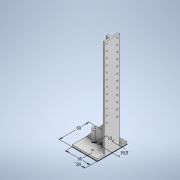
# Autodesk Inventor part: camera arm
Saved by Autodesk Inventor 2021 (Build 250183000, 183)
## iProperties
Created: 2022-11-09
Part Number: camera arm
Material: Generic
Document SubType Name: Modeling
Designer: marti
Density: 1 g/cm^3
Appearance: Default
Author: marti
Autodesk Inventor part; units mm, degrees
ref_plane "YZ Plane" through (0, 0, 0) normal (1, 0, 0) x (0, 1, 0)
ref_plane "XZ Plane" through (0, 0, 0) normal (0, 1, 0) x (-1, 0, 0)
ref_plane "XY Plane" through (0, 0, 0) normal (0, 0, 1) x (1, 0, 0)
sketch "Sketch1" plane through (0, 0, 0) normal (0, 1, 0) x (-1, 0, 0)
  line L0 (-15, -19.5) -> (-15, 0) construction
  line L1 (-15, 0) -> (-15, 19.5) construction
  line L2 (15, -30) -> (-35, -30)
  line L3 (-35, -30) -> (-35, 30)
  line L4 (-35, 30) -> (15, 30)
  line L5 (15, 30) -> (15, -30)
  circle A0 centre (0, 0) radius 5
  point P0 (15, 0)
  dimension "d0" = 15
  dimension "d1" = 19.5
  dimension "d2" = 60
  dimension "d3" = 50
  dimension "d4" = 20
  dimension "d22" = 10
  constraints: 12 end point, 3 equal length, 2 coincident, 2 horizontal alignment, 1 centre point, 1 collinear, 1 horizontal, 1 midpoint, 1 perpendicular, 1 vertical
  measures "d0" horizontal distance of L0.start point (0, 0)
  measures "d1" vertical distance of point (0, 0) L0.start
  measures "d2" distance of L4.end L2.start
  measures "d3" distance of L3.end L4.end
  measures "d4" distance from line of L1.end L3
  measures "d22" diameter of A0
extrude "Extrusion1" add sketch "Sketch1" along normal blind 4 contours L2 L3 L4 L5 | A0
sketch "Sketch2" plane through (0, 0, 0) normal (0, 0, 1) x (1, 0, 0)
  line L0 (35, 4) -> (-15, 4) projected
  line L1 (35, 4) -> (35, 200)
  line L2 (35, 200) -> (25, 200)
  line L3 (25, 200) -> (25, 49)
  line L4 (25, 49) -> (-15, 4)
  line L5 (32, 200) -> (32, 4)
  line L6 (-15, 0) -> (35, 0) projected
  point P0 (0, 0)
  dimension "d14" = 10
  dimension "d15" = 3
  dimension "d16" = 45
  dimension "d17" = 200
  constraints: 10 end point, 3 perpendicular, 2 point on line, 1 vertical
  measures "d14" distance between parallel lines of L3 L1
  measures "d15" distance between parallel lines of L1 L5
  measures "d16" distance from line of L0 L3.end
  measures "d17" distance from line of L6 L5.start
extrude "Extrusion2" add sketch "Sketch2" along normal mid plane 4 contours L0 L4 L3 L2 L5
extrude "breedte arm" add sketch "Sketch2" along normal mid plane 30 contours L0 L5 L2 L1
extrude "Extrusion4" add sketch "Sketch1" along normal blind 25 contours A0
hole "Hole2" at (0, 0, 0) at (15, 0, -19.5) at (15, 0, 19.5) direction (0, 1, 0) diameter 3.4 end through all clearance for "Hex Head Cap Screw ISO 24017" size "M3" standard "ISO"
sketch "Sketch3" plane through (35, 0, 30) normal (1, 0, 0) x (0, 0, -1)
  line L0 (15, 200) -> (45, 200) projected
  line L1 (19.5, 195) -> (15, 195) construction
  line L2 (15, 200) -> (15, 4) construction
  line L3 (40.5, 195) -> (45, 195) construction
  line L4 (45, 4) -> (45, 200) construction
  point P0 (30, 0)
  point P1 (42.75, 195)
  point P2 (19.5, 182.5)
  point P3 (40.5, 182.5)
  point P4 (19.5, 170)
  point P5 (40.5, 170)
  point P6 (19.5, 157.5)
  point P7 (40.5, 157.5)
  point P8 (19.5, 145)
  point P9 (40.5, 145)
  point P10 (19.5, 132.5)
  point P11 (40.5, 132.5)
  point P12 (19.5, 120)
  point P13 (40.5, 120)
  point P14 (19.5, 107.5)
  point P15 (40.5, 107.5)
  point P16 (19.5, 95)
  point P17 (40.5, 95)
  point P18 (19.5, 82.5)
  point P19 (40.5, 82.5)
  point P20 (19.5, 70)
  point P21 (40.5, 70)
  point P22 (19.5, 57.5)
  point P23 (40.5, 57.5)
  dimension "d32" = 5
  dimension "d33" = 21
  dimension "d36" = 12.5
  constraints: 4 end point, 3 point on line, 1 collinear, 1 horizontal, 1 horizontal alignment, 1 midpoint, 1 vertical, 22 other
  measures "d32" distance from line of L1.start L0
  measures "d33" distance of L1.start L3.start
  measures "d36" distance of L1.start point (19.5, 182.5)
hole "Hole3" at (35, 195, 10.5) at (35, 195, -10.5) at (35, 182.5, -10.5) at (35, 182.5, 10.5) at (35, 170, 10.5) at (35, 170, -10.5) at (35, 157.5, -10.5) at (35, 157.5, 10.5) at (35, 145, 10.5) at (35, 145, -10.5) at (35, 132.5, -10.5) at (35, 132.5, 10.5) at (35, 120, 10.5) at (35, 120, -10.5) at (35, 107.5, -10.5) at (35, 107.5, 10.5) at (35, 95, 10.5) at (35, 95, -10.5) at (35, 82.5, 10.5) at (35, 70, 10.5) at (35, 57.5, 10.5) at (35, 57.5, -10.5) at (35, 70, -10.5) at (35, 82.5, -10.5) direction (-1, 0, 0) diameter 2.2 end through all
body "Solid1"
